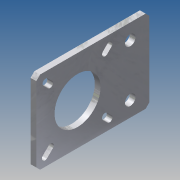
# Autodesk Inventor part: Nema17_Montageplatte_Z-Achse
Saved by Autodesk Inventor 2015 SP1 (Build 190203100, 203)
## iProperties
Created: 2015-01-06
Part Number: Nema17_Montageplatte_Z-Achse
Material: Aluminium 6061
Document SubType Name: Modeling
Designer: Marc
Density: 2.7 g/cm^3
Appearance: Aluminium - flach
Mass: 21.42 g
Surface Area: 62.3386 cm^2
Volume: 7.93335 cm^3
Author: Marc
Autodesk Inventor part; units mm, degrees
ref_plane "YZ Plane" through (0, 0, 0) normal (1, 0, 0) x (0, 1, 0)
ref_plane "XZ Plane" through (0, 0, 0) normal (0, 1, 0) x (-1, 0, 0)
ref_plane "XY Plane" through (0, 0, 0) normal (0, 0, 1) x (1, 0, 0)
sketch "Skizze1" plane through (0, 0, 0) normal (1, 0, 0) x (0, 1, 0)
  line L0 (0, -30.1) -> (0, 30.1) projected
  line L1 (-41.3, 0) -> (41.3, 0) projected
  line L2 (-27.5, 21.5) -> (27.5, 21.5)
  line L3 (29.5, 19.5) -> (29.5, -19.5)
  line L4 (27.5, -21.5) -> (-27.5, -21.5)
  line L5 (-29.5, -19.5) -> (-29.5, 19.5)
  circle A0 centre (19.5, 13.5) radius 2.75
  circle A1 centre (19.5, -13.5) radius 2.75
  line L6 (27.5, 21.5) -> (29.5, 19.5)
  line L7 (29.5, -19.5) -> (27.5, -21.5)
  line L8 (-27.5, 21.5) -> (-29.5, 19.5)
  line L9 (-27.5, -21.5) -> (-29.5, -19.5)
  line L10 (8.6314, 16.6314) -> (6.3686, 14.3686) construction
  line L11 (7.5, 17.7627) -> (5.2373, 15.5)
  line L12 (7.5, 13.2373) -> (9.7627, 15.5)
  arc A2 (9.7627, 15.5) -> (7.5, 17.7627) centre (8.6314, 16.6314) ccw
  arc A3 (5.2373, 15.5) -> (7.5, 13.2373) centre (6.3686, 14.3686) ccw
  line L13 (-24.6314, 16.6314) -> (-22.3686, 14.3686) construction
  line L14 (-25.7627, 15.5) -> (-23.5, 13.2373)
  line L15 (-21.2373, 15.5) -> (-23.5, 17.7627)
  arc A4 (-23.5, 17.7627) -> (-25.7627, 15.5) centre (-24.6314, 16.6314) ccw
  arc A5 (-23.5, 13.2373) -> (-21.2373, 15.5) centre (-22.3686, 14.3686) ccw
  line L16 (8.6314, -16.6314) -> (6.3686, -14.3686) construction
  line L17 (9.7627, -15.5) -> (7.5, -13.2373)
  line L18 (5.2373, -15.5) -> (7.5, -17.7627)
  arc A6 (7.5, -17.7627) -> (9.7627, -15.5) centre (8.6314, -16.6314) ccw
  arc A7 (7.5, -13.2373) -> (5.2373, -15.5) centre (6.3686, -14.3686) ccw
  line L19 (-23.4997, -15.4997) -> (-23.5003, -15.5003) construction
  line L20 (-25.3683, -16.631) -> (-25.369, -16.6317)
  line L21 (-27.6317, -14.369) -> (-27.631, -14.3683)
  line L22 (-24.9849, -16.9849) -> (-22.0151, -14.0151) construction
  line L23 (-23.8536, -18.1163) -> (-20.8837, -15.1464)
  line L24 (-23.1464, -12.8837) -> (-26.1163, -15.8536)
  arc A8 (-26.1163, -15.8536) -> (-23.8536, -18.1163) centre (-24.9849, -16.9849) ccw
  arc A9 (-20.8837, -15.1464) -> (-23.1464, -12.8837) centre (-22.0151, -14.0151) ccw
  circle A10 centre (-8, 0) radius 12
  point P0 (0, 0)
  point P1 (-29.5, 21.5)
  point P2 (29.5, -21.5)
  point P3 (29.5, 21.5)
  point P4 (-29.5, -21.5)
  point P5 (7.5, 15.5)
  point P6 (-23.5, 15.5)
  point P7 (7.5, -15.5)
  point P8 (-23.5, -15.5)
  dimension "d0" = 59
  dimension "d1" = 43
  dimension "d2" = 5.5
  dimension "d3" = 10
  dimension "d4" = 8
  dimension "d14" = 2
  dimension "d15" = 2
  dimension "d16" = 2
  dimension "d17" = 2
  dimension "d18" = 2
  dimension "d19" = 2
  dimension "d20" = 2
  dimension "d21" = 2
  dimension "d22" = 3.2
  dimension "d23" = 3.2
  dimension "d24" = 3.2
  dimension "d26" = 6
  dimension "d27" = 31
  dimension "d28" = 31
  dimension "d31" = 2.1
  dimension "d32" = 3.2
  dimension "d35" = 24
  dimension "d36" = 15.5
  constraints: 56 end point, 19 tangent, 16 point on circle, 11 centre point, 10 point on line, 7 parallel, 5 midpoint, 2 horizontal alignment, 2 perpendicular, 2 vertical alignment, 1 horizontal, 1 symmetric about line, 4 other
  measures "d0" distance of point (29.5, -21.5) point (-29.5, -21.5)
  measures "d1" distance of point (29.5, 21.5) point (29.5, -21.5)
  measures "d2" diameter of A0
  measures "d3" distance from line of L3 A0.centre
  measures "d4" distance from line of L2 A0.centre
  measures "d14" distance of L2.end point (29.5, 21.5)
  measures "d15" distance of L3.start point (29.5, 21.5)
  measures "d16" distance of L3.end point (29.5, -21.5)
  measures "d17" distance of L4.start point (29.5, -21.5)
  measures "d18" distance of L2.start point (-29.5, 21.5)
  measures "d19" distance of L5.end point (-29.5, 21.5)
  measures "d20" distance of L4.end point (-29.5, -21.5)
  measures "d21" distance of L5.start point (-29.5, -21.5)
  measures "d22" diameter of A3
  measures "d23" diameter of A5
  measures "d24" diameter of A7
  measures "d26" distance from line of L5 point (-23.5, -15.5)
  measures "d27" distance of point (-23.5, 15.5) point (-23.5, -15.5)
  measures "d28" distance of point (7.5, -15.5) point (-23.5, -15.5)
  measures "d31" distance of point (-23.5, -15.5) L22.end
  measures "d32" diameter of A9
  measures "d35" diameter of A10
  measures "d36" horizontal distance of point (7.5, -15.5) A10.centre
extrude "Extrusion4" add sketch "Skizze1" along normal mid plane 3 contours L4 L9 L5 L1 A10 L0 | L0 A10 L1 L3 L7 L4 | L1 L5 L8 L2 L0 A10 | A10 L0 L2 L6 L3 L1
equation "\"d15\" = d14"
equation "\"d16\" = d14"
equation "\"d17\" = d16"
equation "\"d18\" = d14"
equation "\"d19\" = d18"
equation "\"d20\" = d14"
equation "\"d21\" = d20"
